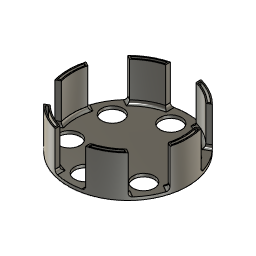
v01.01-sim-dash-g920-base (Autodesk Fusion 360 design; units mm, degrees)
Autodesk Fusion 360 part; units mm, degrees
sketch "Sketch1" plane through (0, 0, 0) normal (0, 0, 1) x (1, 0, 0)
  circle A0 centre (0, 0) radius 39
  dimension "d5" = 78
  constraint coincident A0.centre origin
  measures "d5" diameter of A0
extrude "Extrude1" add sketch "Sketch1" along normal blind 2
sketch "Sketch4" plane through (0, 0, 2) normal (0, 0, 1) x (-1, 0, 0)
  circle A0 centre (0, 0) radius 39
  circle A1 centre (0, 0) radius 36
  circle A2 centre (0, 0) radius 39
  dimension "d7" = 78
  dimension "d8" = 72
  constraint concentric A0 A1
  constraint concentric A1 A2
  measures "d7" diameter of A2
  measures "d8" diameter of A1
extrude "Extrude3" add sketch "Sketch4" along normal blind 25
sketch "Sketch8" plane through (0, 0, 2) normal (0, 0, 1) x (-1, 0, 0)
  circle A0 centre (0, 28) radius 7
  circle A1 centre (-24.2487, 14) radius 7
  circle A2 centre (-24.2487, -14) radius 7
  circle A3 centre (0, -28) radius 7
  circle A4 centre (24.2487, -14) radius 7
  circle A5 centre (24.2487, 14) radius 7
  dimension "d26" = 14
  dimension "d28" = 360
  dimension "d29" = 28
  constraint vertical A0.centre origin
  measures "d26" diameter of A0
  measures "d29" vertical distance of A0.centre origin
extrude "Extrude6" cut sketch "Sketch8" against normal through all
sketch "Sketch6" plane through (0, 0, 27) normal (0, 0, 1) x (-1, 0, 0)
  circle A0 centre (0, 0) radius 36
  circle A1 centre (0, 0) radius 39
  line L0 (10, 12.5455) -> (-10, 12.5455)
  line L1 (-10, 12.5455) -> (-10, 52.5455)
  line L2 (-10, 52.5455) -> (10, 52.5455)
  line L3 (10, 52.5455) -> (10, 12.5455)
  line L4 (-40.5057, 34.933) -> (-5.8647, 14.933)
  line L5 (-50.5057, 17.6125) -> (-40.5057, 34.933)
  line L6 (-15.8647, -2.3875) -> (-50.5057, 17.6125)
  line L7 (-50.5057, -17.6125) -> (-15.8647, 2.3875)
  line L8 (-40.5057, -34.933) -> (-50.5057, -17.6125)
  line L9 (-5.8647, -14.933) -> (-40.5057, -34.933)
  line L10 (-10, -52.5455) -> (-10, -12.5455)
  line L11 (10, -52.5455) -> (-10, -52.5455)
  line L12 (10, -12.5455) -> (10, -52.5455)
  line L13 (40.5057, -34.933) -> (5.8647, -14.933)
  line L14 (50.5057, -17.6125) -> (40.5057, -34.933)
  line L15 (15.8647, 2.3875) -> (50.5057, -17.6125)
  line L16 (50.5057, 17.6125) -> (15.8647, -2.3875)
  line L17 (40.5057, 34.933) -> (50.5057, 17.6125)
  line L18 (5.8647, 14.933) -> (40.5057, 34.933)
  dimension "d11" = 20
  dimension "d12" = 40
  dimension "d13" = 10
  dimension "d33" = 360
  constraint horizontal L0
  constraint vertical L1
  constraint horizontal L2
  constraint vertical L3
  measures "d11" distance of L0.start L0.end
  measures "d12" distance of L0.start L2.end
  measures "d13" distance of A0.centre L3
extrude "Extrude7" cut sketch "Sketch6" against normal up to surface (25 mm away) contours A0 A1 L16 L18 | A0 A1 L13 L15 | A0 A1 L1 L3 | A0 A1 L10 L12 | A0 A1 L4 L6 | A0 A1 L7 L9
sketch "Sketch9" plane through (0, 0, 27) normal (0, 0, 1) x (-1, 0, 0)
  line L0 (27.6458, -27.5083) -> (24.95, -25.9519)
  arc A0 (10, -34.5832) -> (24.95, -25.9519) centre (0, 0) ccw
  line L1 (10, -34.5832) -> (10, -37.6962)
  arc A1 (10, -37.6962) -> (27.6458, -27.5083) centre (0, 0) ccw
  circle A2 centre (0, 0) radius 38.25
  circle A3 centre (0, 0) radius 36.75
  line L2 (11, -45) -> (-11, -45)
  line L3 (-11, -45) -> (-11, -19)
  line L4 (-11, -19) -> (11, -19)
  line L5 (11, -19) -> (11, -45)
  line L6 (44.4711, -12.9737) -> (33.4711, -32.0263)
  line L7 (21.9545, 0.0263) -> (44.4711, -12.9737)
  line L8 (10.9545, -19.0263) -> (21.9545, 0.0263)
  line L9 (33.4711, -32.0263) -> (10.9545, -19.0263)
  line L10 (33.4711, 32.0263) -> (44.4711, 12.9737)
  line L11 (10.9545, 19.0263) -> (33.4711, 32.0263)
  line L12 (21.9545, -0.0263) -> (10.9545, 19.0263)
  line L13 (44.4711, 12.9737) -> (21.9545, -0.0263)
  line L14 (-11, 45) -> (11, 45)
  line L15 (-11, 19) -> (-11, 45)
  line L16 (11, 19) -> (-11, 19)
  line L17 (11, 45) -> (11, 19)
  line L18 (-44.4711, 12.9737) -> (-33.4711, 32.0263)
  line L19 (-21.9545, -0.0263) -> (-44.4711, 12.9737)
  line L20 (-10.9545, 19.0263) -> (-21.9545, -0.0263)
  line L21 (-33.4711, 32.0263) -> (-10.9545, 19.0263)
  line L22 (-33.4711, -32.0263) -> (-44.4711, -12.9737)
  line L23 (-10.9545, -19.0263) -> (-33.4711, -32.0263)
  line L24 (-21.9545, 0.0263) -> (-10.9545, -19.0263)
  line L25 (-44.4711, -12.9737) -> (-21.9545, 0.0263)
  dimension "d36" = 76.5
  dimension "d37" = 73.5
  dimension "d38" = 22
  dimension "d39" = 11
  dimension "d41" = 360
  constraint concentric A0 A2
  constraint concentric A2 A3
  constraint horizontal L2
  constraint vertical L3
  constraint horizontal L4
  constraint vertical L5
  measures "d36" diameter of A2
  measures "d37" diameter of A3
  measures "d38" distance of L2.start L2.end
  measures "d39" horizontal distance of A0.centre L4.end
extrude "Extrude8" cut sketch "Sketch9" against normal up to surface (25 mm away) contours A2 A3 L5 L9 | A2 A3 L7 L13 | A2 A3 L3 L23 | A2 A3 L11 L17 | A2 A3 L19 L25 | A2 A3 L15 L21
fillet "Fillet3" radius 2 18 edges at (-36, 0, 2) (-18, 31.1769, 2) (-36.2979, -9.4096, 2) (-36.2979, 9.4096, 2) (-10, 36.1397, 2) (-26.2979, 26.7301, 2) (18, 31.1769, 2) (26.2979, 26.7301, 2) (10, 36.1397, 2) (36.2979, 9.4096, 2) (36, 0, 2) (36.2979, -9.4096, 2) (10, -36.1397, 2) (18, -31.1769, 2) (26.2979, -26.7301, 2) (-18, -31.1769, 2) (-26.2979, -26.7301, 2) (-10, -36.1397, 2)
